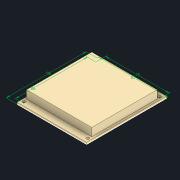
# Autodesk Inventor part: mainboard
Saved by Autodesk Inventor 2022 (Build 260153000, 153)
## iProperties
Created: 2022-01-04
Part Number: mainboard
Material: Generic
Document SubType Name: Modeling
Designer: Andres
Density: 1 g/cm^3
Appearance: Beige
Author: Andres
Autodesk Inventor part; units mm, degrees
ref_plane "YZ Plane" through (0, 0, 0) normal (1, 0, 0) x (0, 1, 0)
ref_plane "XZ Plane" through (0, 0, 0) normal (0, 1, 0) x (-1, 0, 0)
ref_plane "XY Plane" through (0, 0, 0) normal (0, 0, 1) x (1, 0, 0)
sketch "Sketch1" plane through (0, 0, 0) normal (0, 1, 0) x (-1, 0, 0)
  line L0 (-42.5, 49) -> (42.5, 49)
  line L1 (42.5, 49) -> (42.5, -49)
  line L2 (42.5, -49) -> (-42.5, -49)
  line L3 (-42.5, -49) -> (-42.5, 49)
  line L4 (-42.5, 49) -> (42.5, -49) construction
  line L5 (42.5, 49) -> (-42.5, -49) construction
  line L6 (-39, 44) -> (39, 44) construction
  line L7 (39, 44) -> (39, -44) construction
  line L8 (39, -44) -> (-39, -44) construction
  line L9 (-39, -44) -> (-39, 44) construction
  line L10 (-39, 44) -> (39, -44) construction
  line L11 (39, 44) -> (-39, -44) construction
  point P0 (0, 0)
  dimension "d0" = 85
  dimension "d1" = 98
  dimension "d2" = 78
  dimension "d3" = 88
  constraints: 24 end point, 4 coincident, 4 midpoint, 4 parallel, 2 horizontal, 2 perpendicular
  measures "d0" distance of L1.end L2.end
  measures "d1" distance of L0.end L1.end
  measures "d2" distance of L7.end L8.end
  measures "d3" distance of L6.end L7.end
extrude "Extrusion1" add sketch "Sketch1" along normal blind 2
hole "Hole1" at (39, 0, 44) at (39, 0, -44) at (-39, 0, -44) at (-39, 0, 44) direction (0, 1, 0) diameter 3.6 end through all clearance for "Socket Head Cap Screw ISO 4762" size "M3" standard "ISO"
sketch "Sketch2" plane through (0, 2, 0) normal (0, 1, 0) x (1, 0, 0)
  line L0 (40, -40) -> (-40, -40)
  line L1 (-40, -40) -> (-40, 40)
  line L2 (-40, 40) -> (40, 40)
  line L3 (40, 40) -> (40, -40)
  line L4 (40, -40) -> (-40, 40) construction
  line L5 (-40, -40) -> (40, 40) construction
  point P0 (0, 0)
  dimension "d13" = 80
  dimension "d14" = 80
  constraints: 12 end point, 2 midpoint, 2 parallel, 1 horizontal, 1 perpendicular
  measures "d13" distance of L1.end L2.end
  measures "d14" distance of L0.end L1.end
extrude "Extrusion2" add sketch "Sketch2" along normal blind 10
body "Solid1"
